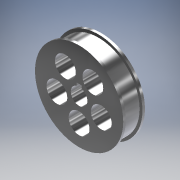
# Autodesk Inventor part: HTD5M 50 Pulley
Saved by Autodesk Inventor 2019.4 (Build 234330000, 330)
## iProperties
Created: 2019-12-31
Part Number: HTD5M 50 Pulley
Material: Aluminum 6061
Document SubType Name: Modeling
Designer: Mark
Mass: 190.325 g
Surface Area: 222.82 cm^2
Volume: 70.4906 cm^3
Density: 2.7 g/cm^3
Appearance: Aluminum - Flat
Author: Mark
Autodesk Inventor part; units mm, degrees
ref_plane "YZ Plane" through (0, 0, 0) normal (1, 0, 0) x (0, 1, 0)
ref_plane "XZ Plane" through (0, 0, 0) normal (0, 1, 0) x (-1, 0, 0)
ref_plane "XY Plane" through (0, 0, 0) normal (0, 0, 1) x (1, 0, 0)
sketch "Sketch1" plane through (0, 0, 0) normal (0, 0, 1) x (1, 0, 0)
  circle A0 centre (0, 0) radius 42.5
  dimension "d0" = 85
  constraints: 1 centre point, 1 coincident
  measures "d0" diameter of A0
extrude "Extrusion1" add sketch "Sketch1" along normal blind 2.5
sketch "Sketch2" plane through (0, 0, 2.5) normal (0, 0, 1) x (1, 0, 0)
  circle A0 centre (0, 0) radius 39.79
  dimension "d3" = 79.58
  constraints: 1 centre point, 1 coincident
  measures "d3" diameter of A0
extrude "Extrusion2" add sketch "Sketch2" along normal blind 16
sketch "Sketch3" plane through (0, 0, 18.5) normal (0, 0, 1) x (1, 0, 0)
  circle A0 centre (0, 0) radius 42.5
  dimension "d6" = 85
  constraints: 1 centre point, 1 coincident
  measures "d6" diameter of A0
extrude "Extrusion3" add sketch "Sketch3" along normal blind 2.5
sketch "Sketch4" plane through (0, 0, 21) normal (0, 0, 1) x (1, 0, 0)
  circle A0 centre (0, 0) radius 8
  line L0 (-2.5, 5.7) -> (2.5, 5.7)
  line L1 (2.5, 5.7) -> (2.5, 10.3)
  line L2 (2.5, 10.3) -> (-2.5, 10.3)
  line L3 (-2.5, 10.3) -> (-2.5, 5.7)
  line L4 (-2.5, 5.7) -> (2.5, 10.3) construction
  line L5 (2.5, 5.7) -> (-2.5, 10.3) construction
  circle A1 centre (0, 0) radius 22.5
  circle A2 centre (0, -22.5) radius 10
  line L6 (0, 0) -> (0, -22.5)
  line L7 (0, 0) -> (22.5, 0) construction
  circle A3 centre (21.3988, -6.9529) radius 10
  circle A4 centre (13.2252, 18.2029) radius 10
  circle A5 centre (-13.2252, 18.2029) radius 10
  circle A6 centre (-21.3988, -6.9529) radius 10
  point P0 (0, 8)
  dimension "d9" = 16
  dimension "d14" = 45
  dimension "d10" = 5
  dimension "d11" = 4.6
  dimension "d15" = 20
  dimension "d16" = 90
  dimension "d19" = 360
  constraints: 16 end point, 5 centre point, 2 coincident, 2 horizontal, 2 midpoint, 2 parallel, 2 perpendicular, 2 vertical alignment, 15 other
  measures "d10" distance of L2.end L1.end
  measures "d11" distance of L1.end L0.end
  measures "d15" diameter of A2
  measures "d16" angle of L6 L7
extrude "Extrusion4" cut sketch "Sketch4" against normal blind 21 contours A0 L3 L0 L1 | A2 A1 L6 | L6 A1 A2 | L1 L0 L3 A0 | A0 L3 L2 L1 | A2 A1 | A3 A1 | A1 A3 | A6 A1 | A1 A6 | A4 A1 | A1 A4 | A5 A1 | A1 A5
body "Solid1"
